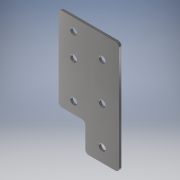
# Autodesk Inventor part: Oxy_cut
Saved by Autodesk Inventor 2019 (Build 230136000, 136)
## iProperties
Created: 2021-02-03
Part Number: Oxy_cut
Material: Stainless Steel
Document SubType Name: Modeling
Designer: rtavi
Density: 8 g/cm^3
Appearance: Semi-Polished
Mass: 24.5922 g
Surface Area: 45.147 cm^2
Volume: 3.07403 cm^3
Author: rtavi
Autodesk Inventor part; units mm, degrees
ref_plane "YZ Plane" through (0, 0, 0) normal (1, 0, 0) x (0, 1, 0)
ref_plane "XZ Plane" through (0, 0, 0) normal (0, 1, 0) x (-1, 0, 0)
ref_plane "XY Plane" through (0, 0, 0) normal (0, 0, 1) x (1, 0, 0)
sketch "Sketch2" plane through (0, 0, 0) normal (0, 0, 1) x (1, 0, 0)
  arc A0 (93, -22.6) -> (97, -22.6) centre (95, -22.6) ccw construction
  arc A1 (97, -22.6) -> (93, -22.6) centre (95, -22.6) ccw construction
  arc A2 (97, 22.6) -> (93, 22.6) centre (95, 22.6) ccw construction
  arc A3 (93, 22.6) -> (97, 22.6) centre (95, 22.6) ccw construction
  line L0 (207.9, 0) -> (-207.9, 0) construction
  line L1 (0, -294.0706) -> (0, 294.0706) construction
  line L2 (87, -30.6) -> (103, -30.6)
  line L3 (105, -28.6) -> (105, 34)
  line L4 (103, 36) -> (71, 36)
  line L5 (69, 34) -> (69, -12)
  line L6 (71, -14) -> (83, -14)
  line L7 (85, -16) -> (85, -28.6)
  arc A4 (103, -30.6) -> (105, -28.6) centre (103, -28.6) ccw
  arc A5 (85, -28.6) -> (87, -30.6) centre (87, -28.6) ccw
  arc A6 (85, -16) -> (83, -14) centre (83, -16) ccw
  arc A7 (69, -12) -> (71, -14) centre (71, -12) ccw
  arc A8 (71, 36) -> (69, 34) centre (71, 34) ccw
  arc A9 (105, 34) -> (103, 36) centre (103, 34) ccw
  circle A10 centre (78, -7.2) radius 2.05
  circle A11 centre (78, 14.8) radius 2.05
  circle A12 centre (78, 28.8) radius 2.05
  line L8 (78, -7.2) -> (78, 28.8) construction
  line L9 (98, -18.65) -> (98, -26.55) construction
  line L10 (98, -26.55) -> (92, -26.55) construction
  line L11 (92, -18.65) -> (92, -26.55) construction
  line L12 (98, -18.65) -> (92, -18.65) construction
  arc A13 (97, -22.6) -> (93, -22.6) centre (95, -22.6) ccw construction
  arc A14 (93, -22.6) -> (97, -22.6) centre (95, -22.6) ccw construction
  line L13 (92, 18.65) -> (92, 26.55) construction
  line L14 (92, 26.55) -> (98, 26.55) construction
  line L15 (98, 18.65) -> (98, 26.55) construction
  line L16 (92, 18.65) -> (98, 18.65) construction
  arc A15 (93, 22.6) -> (97, 22.6) centre (95, 22.6) ccw construction
  arc A16 (97, 22.6) -> (93, 22.6) centre (95, 22.6) ccw construction
  arc A17 (97, -22.6) -> (93, -22.6) centre (95, -22.6) ccw construction
  arc A18 (97.4356, -1.2768) -> (97.4356, 1.2768) centre (95, 0) ccw construction
  circle A19 centre (95, 0) radius 2.05
  circle A20 centre (95, 22.6) radius 2.05
  circle A21 centre (95, -22.6) radius 2.05
  point P0 (0, 0)
  point P1 (105, 36)
  point P2 (69, 36)
extrude "Extrusion2" add sketch "Sketch2" along normal blind 1.5
body "Solid2"
